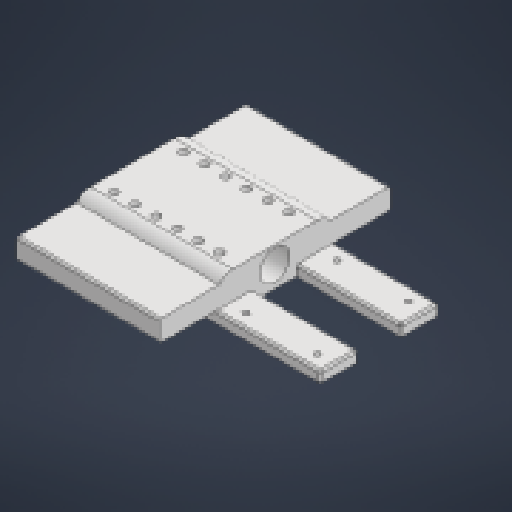
# Autodesk Inventor part: Tourniquet_Rail_01_V4
Saved by Autodesk Inventor 2026.2 (Build 302298000, 298)
## iProperties
Created: 2026-03-17
Part Number: Tourniquet_Rail_01_V4
Material: Generic
Document SubType Name: Modeling
Designer: vckot
Density: 1 g/cm^3
Appearance: Default
Author: vckot
Autodesk Inventor part; units mm, degrees
ref_plane "YZ Plane" through (0, 0, 0) normal (1, 0, 0) x (0, 1, 0)
ref_plane "XZ Plane" through (0, 0, 0) normal (0, 1, 0) x (-1, 0, 0)
ref_plane "XY Plane" through (0, 0, 0) normal (0, 0, 1) x (1, 0, 0)
sketch "Sketch1" plane through (0, 0, 0) normal (1, 0, 0) x (0, 1, 0)
  circle A0 centre (0, 0) radius 3.625
  line L0 (-5, 0) -> (5, 0) construction
  line L1 (-2.5, 14.125) -> (-2.5, 27.5)
  line L2 (-2.5, 27.5) -> (2.5, 27.5)
  line L3 (2.5, 27.5) -> (2.5, 13.2811)
  line L4 (-2.5, -14.125) -> (-2.5, -27.5)
  line L5 (-2.5, -27.5) -> (2.5, -27.5)
  line L6 (2.5, -27.5) -> (2.5, -13.2811)
  line L7 (-5, -14.125) -> (-5, 14.125)
  line L8 (0, -14.125) -> (-5, -14.125)
  arc A1 (0, -14.125) -> (4.125, -10) centre (0, -10) ccw
  line L9 (4.125, 10) -> (4.125, -10)
  arc A2 (4.125, 10) -> (0, 14.125) centre (0, 10) ccw
  line L10 (-5, 14.125) -> (0, 14.125)
  point P0 (4.125, 0)
  point P1 (-2.5, 20.8125)
  point P2 (-2.5, 14.125)
  point P3 (-2.5, -20.8125)
  point P4 (-2.5, -14.125)
  dimension "d0" = 7.25
  dimension "d8" = 10
  dimension "d9" = 5
  dimension "d10" = 5
  dimension "d11" = 27.5
  dimension "d12" = 27.5
  dimension "d17" = 9.125
  dimension "d18" = 28.25
  dimension "d19" = 4.125
  dimension "d20" = 4.125
  dimension "d21" = 5
  dimension "d22" = 14.125
  constraints: 22 end point, 8 midpoint, 6 point on circle, 5 perpendicular, 4 tangent, 3 centre point, 2 horizontal alignment, 2 vertical, 2 vertical alignment, 1 coincident, 1 horizontal
  measures "d0" diameter of A0
  measures "d8" distance of L0.start L0.end
  measures "d9" distance of L1.end L2.end
  measures "d10" distance between parallel lines of L4 L6
  measures "d11" distance from line of L2 A0.centre
  measures "d12" distance from line of L5 A0.centre
  measures "d17" distance between parallel lines of L7 L9
  measures "d18" distance between parallel lines of L8 L10
  measures "d19" radius of A2
  measures "d20" radius of A1
  measures "d21" distance from line of A0.centre L7
  measures "d22" distance from line of L8 A0.centre
extrude "Extrusion1" add sketch "Sketch1" along normal blind 34
sketch "Sketch2" plane through (0, 4.125, 10) normal (0, 1, 0) x (1, 0, 0)
  line L0 (0, 20) -> (0, 0) projected
  line L1 (0, -3.2811) -> (34, -3.2811) projected
  line L2 (0, 10) -> (34, 10) construction
  line L3 (34, 20) -> (34, 0) construction
  point P0 (4, 1.7189)
  point P1 (4, 18.2811)
  dimension "d23" = 4
  dimension "d24" = 5
  constraints: 2 end point, 1 midpoint, 1 symmetric about line
  measures "d23" distance from line of point (4, 1.719) L0
  measures "d24" distance from line of L1 point (4, 1.719)
hole "Hole1" at (4, 4.125, 8.2811) at (4, 4.125, -8.2811) direction (0, -1, 0) diameter 2 end through all
pattern_linear "Rectangular Pattern1" count 6 spacing 5 along (1, 0, 0) of "Hole1"
sketch "Sketch3" plane through (34, 0, 0) normal (1, 0, 0) x (0, 0, -1)
  line L0 (-14.125, -5) -> (14.125, -5) projected
  line L1 (-14.125, -5) -> (-5.125, -5)
  line L2 (-5.125, -5) -> (-5.125, -2.5)
  line L3 (-5.125, -2.5) -> (-14.125, -2.5)
  line L4 (-14.125, -2.5) -> (-14.125, -5)
  line L5 (14.125, -5) -> (5.125, -5)
  line L6 (5.125, -5) -> (5.125, -2.5)
  line L7 (5.125, -2.5) -> (14.125, -2.5)
  line L8 (14.125, -2.5) -> (14.125, -5)
  point P0 (0, 0)
  dimension "d35" = 9
  dimension "d36" = 2.5
  dimension "d37" = 9
  dimension "d38" = 2.5
  constraints: 16 end point, 4 parallel, 2 horizontal, 2 perpendicular
  measures "d35" distance of L3.end L2.end
  measures "d36" distance of L2.end L1.end
  measures "d37" distance of L6.end L7.end
  measures "d38" distance of L5.end L6.end
extrude "Extrusion2" add sketch "Sketch3" along normal blind 25
sketch "Sketch4" plane through (34, -2.5, 14.125) normal (0, 1, 0) x (1, 0, 0)
  line L0 (21, 3.25) -> (4, 3.25) construction
  line L1 (21, 25) -> (4, 25) construction
  line L2 (0, 19.25) -> (25, 19.25) construction
  line L3 (0, 9) -> (25, 9) construction
  line L4 (25, 9) -> (25, 0) construction
  line L5 (25, 28.25) -> (25, 19.25) construction
  circle A0 centre (21, -4.25) radius 0.75 projected
  circle A1 centre (4, -4.25) radius 0.75 projected
  circle A2 centre (21, 32.5) radius 0.75 projected
  circle A3 centre (4, 32.5) radius 0.75 projected
  point P0 (-34, 14.125)
  point P1 (12.5, 25)
  point P2 (12.5, 19.25)
  point P3 (12.5, 3.25)
  point P4 (12.5, 9)
  dimension "d48" = 17
  dimension "d49" = 17
  dimension "d50" = 7.5
  dimension "d51" = 7.5
  constraints: 4 end point, 4 midpoint, 2 horizontal, 2 horizontal alignment, 2 vertical alignment
  measures "d48" distance of L0.start L0.end
  measures "d49" distance of L1.end L1.start
  measures "d50" distance of A2.centre L1.start
  measures "d51" distance of A0.centre L0.start
hole "Hole2" at (38, -2.5, 10.875) at (55, -2.5, 10.875) at (55, -2.5, -10.875) at (38, -2.5, -10.875) direction (0, -1, 0) diameter 1.5 end through all
fillet "Fillet1" radius 0.5 10 edges at (46.5, -2.5, 14.125) (59, -3.75, 14.125) (59, -2.5, 9.625) (59, -3.75, 5.125) (46.5, -2.5, 5.125) (46.5, -2.5, -5.125) (59, -3.75, -5.125) (59, -2.5, -9.625) (59, -3.75, -14.125) (46.5, -2.5, -14.125)
fillet "Fillet2" radius 0.5 4 edges at (17, 2.5, -27.5) (17, -2.5, -27.5) (17, 2.5, 27.5) (17, -2.5, 27.5)
body "Solid1"
